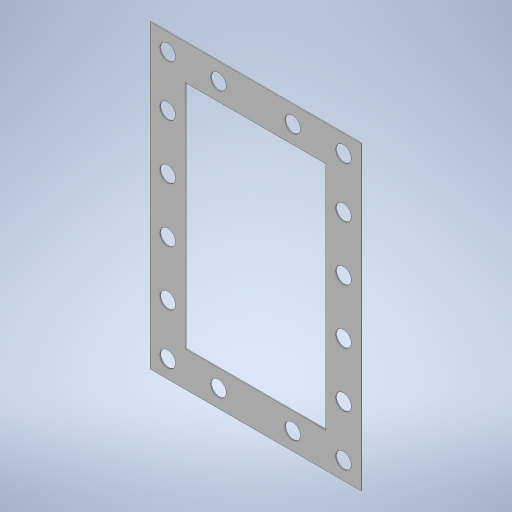
# Autodesk Inventor part: HUDSON-1-34
Saved by Autodesk Inventor 2024.2 (Build 282272000, 272)
## iProperties
Created: 2024-11-02
Part Number: HUDSON-1-34
Material: Generic
Document SubType Name: Modeling
Designer: melim
Density: 1 g/cm^3
Appearance: Default
Author: melim
Autodesk Inventor part; units mm, degrees
ref_plane "YZ Plane" through (0, 0, 0) normal (1, 0, 0) x (0, 1, 0)
ref_plane "XZ Plane" through (0, 0, 0) normal (0, 1, 0) x (-1, 0, 0)
ref_plane "XY Plane" through (0, 0, 0) normal (0, 0, 1) x (1, 0, 0)
sketch "Sketch1" plane through (0, 0, 0) normal (0, 0, 1) x (1, 0, 0)
  line L0 (27, 38.5) -> (-27, 38.5)
  line L1 (-27, 38.5) -> (-27, -38.5)
  line L2 (-27, -38.5) -> (27, -38.5)
  line L3 (27, -38.5) -> (27, 38.5)
  line L4 (27, 38.5) -> (-27, -38.5) construction
  line L5 (-27, 38.5) -> (27, -38.5) construction
  line L6 (-18, 29.5) -> (18, 29.5)
  line L7 (18, 29.5) -> (18, -29.5)
  line L8 (18, -29.5) -> (-18, -29.5)
  line L9 (-18, -29.5) -> (-18, 29.5)
  line L10 (-27, 0) -> (27, 0)
  line L11 (0, 38.5) -> (0, -38.5)
  point P0 (0, 0)
  point P1 (0, 29.5)
  point P2 (-22.5, 34)
  point P3 (-9.5, 34)
  point P4 (9.5, 34)
  point P5 (22.5, 34)
  point P6 (-22.5, -34)
  point P7 (-9.5, -34)
  point P8 (9.5, -34)
  point P9 (22.5, -34)
  point P10 (-22.5, 21)
  point P11 (-22.5, 7)
  point P12 (-22.5, -21)
  point P13 (-22.5, -7)
  point P14 (22.5, 21)
  point P15 (22.5, 7)
  point P16 (22.5, -21)
  point P17 (22.5, -7)
  dimension "d0" = 77
  dimension "d1" = 54
  dimension "d2" = 59
  dimension "d3" = 36
  dimension "d4" = 18
  dimension "d5" = 29.5
  dimension "d6" = 4.5
  dimension "d7" = 4.5
  dimension "d8" = 4.5
  dimension "d9" = 4.5
  dimension "d10" = 13
  dimension "d11" = 13
  dimension "d12" = 4.5
  dimension "d13" = 4.5
  dimension "d14" = 4.5
  dimension "d15" = 13
  dimension "d16" = 13
  dimension "d17" = 4.5
  dimension "d18" = 14
  dimension "d19" = 14
  dimension "d20" = 4.5
  dimension "d21" = 4.5
  constraints: 24 end point, 8 symmetric about line, 7 midpoint, 4 parallel, 2 horizontal, 2 perpendicular
  measures "d0" distance of L0.end L1.end
  measures "d1" distance of L0.start L0.end
  measures "d2" distance of L6.end L7.end
  measures "d3" distance of L6.start L6.end
  measures "d4" distance from line of L9 point (0, 0)
  measures "d5" distance of point (0, 29.5) point (0, 0)
  measures "d6" distance from line of L3 point (22.5, 34)
  measures "d7" distance from line of L0 point (22.5, 34)
  measures "d8" distance from line of L1 point (-22.5, 34)
  measures "d9" distance from line of L0 point (-22.5, 34)
  measures "d10" distance of point (-22.5, 34) point (-9.5, 34)
  measures "d11" distance of point (22.5, 34) point (9.5, 34)
  measures "d12" distance from line of L0 point (9.5, 34)
  measures "d13" distance from line of L0 point (-9.5, 34)
  measures "d14" distance from line of L1 point (-22.5, 21)
  measures "d15" distance of point (-22.5, 34) point (-22.5, 21)
  measures "d16" distance of point (-22.5, -34) point (-22.5, -21)
  measures "d17" distance from line of L1 point (-22.5, -21)
  measures "d18" distance of point (-22.5, 21) point (-22.5, 7)
  measures "d19" distance of point (-22.5, -7) point (-22.5, 7)
  measures "d20" distance from line of L1 point (-22.5, 7)
  measures "d21" distance from line of L1 point (-22.5, -7)
extrude "Extrusion1" add sketch "Sketch1" along normal blind 0.2 contours L3 L10 L7 L6 L11 L0 | L11 L6 L9 L10 L1 L0 | L3 L2 L11 L8 L7 L10 | L10 L9 L8 L11 L2 L1
hole "Hole1" at (-22.5, 34, 0) at (-9.5, 34, 0) at (9.5, 34, 0) at (22.5, 34, 0) at (-22.5, -34, 0) at (-9.5, -34, 0) at (9.5, -34, 0) at (22.5, -34, 0) at (-22.5, 21, 0) at (-22.5, 7, 0) at (-22.5, -21, 0) at (-22.5, -7, 0) at (22.5, 21, 0) at (22.5, 7, 0) at (22.5, -7, 0) at (22.5, -21, 0) direction (0, 0, 1) diameter 4 end through all
body "Solid1"
